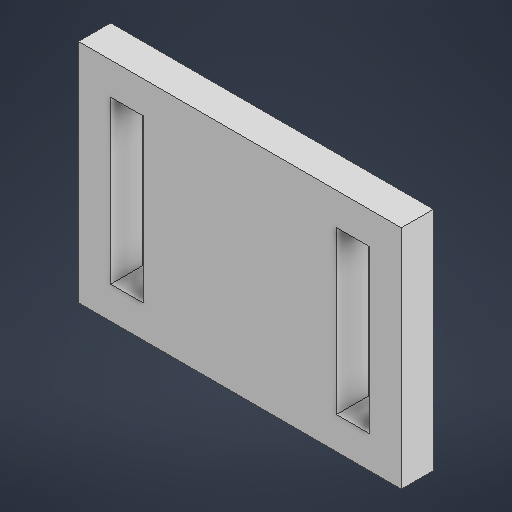
# Autodesk Inventor part: holder
Saved by Autodesk Inventor 2027 (Build 310192000, 192)
## iProperties
Created: 2026-06-03
Part Number: holder
Material: Generic
Document SubType Name: Modeling
Designer: alexy
Density: 1 g/cm^3
Appearance: Default
Author: alexy
Autodesk Inventor part; units mm, degrees
ref_plane "YZ Plane" through (0, 0, 0) normal (1, 0, 0) x (0, 1, 0)
ref_plane "XZ Plane" through (0, 0, 0) normal (0, 1, 0) x (-1, 0, 0)
ref_plane "XY Plane" through (0, 0, 0) normal (0, 0, 1) x (1, 0, 0)
sketch "Sketch1" plane through (0, 0, 0) normal (0, 0, 1) x (1, 0, 0)
  line L0 (0, 21.1) -> (30.1, 21.1)
  line L1 (30.1, 21.1) -> (30.1, 0)
  line L2 (30.1, 0) -> (0, 0)
  line L3 (0, 0) -> (0, 21.1)
  line L4 (3, 18.1) -> (6.05, 18.1)
  line L5 (6.05, 18.1) -> (6.05, 3)
  line L6 (6.05, 3) -> (3, 3)
  line L7 (3, 3) -> (3, 18.1)
  line L8 (24.05, 18.1) -> (27.1, 18.1)
  line L9 (27.1, 18.1) -> (27.1, 3)
  line L10 (27.1, 3) -> (24.05, 3)
  line L11 (24.05, 3) -> (24.05, 18.1)
  dimension "d2" = 3.05
  dimension "d3" = 3.05
  dimension "d4" = 15.1
  dimension "d5" = 18
  dimension "d7" = 3
  dimension "d8" = 3
  dimension "d9" = 3
  dimension "d10" = 3
  constraints: 24 end point, 6 parallel, 3 horizontal, 3 perpendicular, 1 coincident, 1 horizontal alignment, 1 point on line
  measures "d2" distance of L4.start L4.end
  measures "d3" distance of L8.start L8.end
  measures "d4" distance of L4.end L5.end
  measures "d5" distance between parallel lines of L11 L5
  measures "d7" horizontal distance of L8.end L0.end
  measures "d8" distance from line of L2 L9.end
  measures "d9" horizontal distance of L0.start L4.start
  measures "d10" horizontal distance of L0.end L8.end
extrude "Extrusion1" add sketch "Sketch1" along normal blind 3
body "Solid1"
